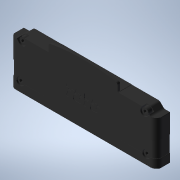
# Autodesk Inventor part: ETH2-17-L_2
Saved by Autodesk Inventor 2021 (Build 250183000, 183)
## iProperties
Created: 2025-05-01
Part Number: ETH2-17-L_2
Material: Generic
Catalog Web Link: www.cadenas.de
Description: ETH2_17_2-ETH2
Vendor: TOYO
Document SubType Name: Modeling
Designer: psAdmin
Manufacturer: TOYO
Mass: 101.271 g
Surface Area: 224.484 cm^2
Volume: 101.271 cm^3
Density: 1 g/cm^3
Appearance: PSOLRGB-175-175-175
Category: PARTsolutions
Company: TOYO
Title: ETH2-17-L
Author: Cadenas PARTsolutions
Comments: ETH2
PSOL_IDENT_0: {$CADENAS_DATA/23d-libs/toyo/eth2_series/eth2_17/parts/eth2_17_body2.prj},165 {VTYP=3D},{NB=ETH2-17-
PSOL_IDENT_1: L_2},{LINA=ETH2-17-L},{NN=ETH2_17_2},{DATE=02.07.2024 05:59:00},{GEOMDATE=07.06.2024 03:32:00},{VERS
PSOL_IDENT_2: ION=},{LINEID=10},{WBVAR=SD},{WBNUMERIC=}  {NB=ETH2-17-L_2},{LINA=ETH2-17-L},{KT=DUMMY},{CNSORDERNO=
PSOL_IDENT_3: ETH2-17-L},{MODEL=ETH2-17},{SD=L}
NB: ETH2-17-L_2
NN: ETH2_17_2
NT: ETH2
NBSYN: $CNSORDERNO._2
LINA: ETH2-17-L
CATALOG: TOYO
MODEL: ETH2-17
SD: L: Left side of slide
SUPPLIER: TOYO
ARTICLENO: ETH2-17-L_2
BOMINFO: ETH2-17-L
CREATOR: CADENAS GmbH
Autodesk Inventor part; units mm, degrees
sketch "__7" plane through (0, 0, 0) normal (0, 0, 1) x (1, 0, 0)
  arc A0 (-75.05, 41.2828) -> (-74.9914, 41.1414) centre (-74.85, 41.2828) ccw
  line L0 (-74.9914, 41.1414) -> (-74.6814, 40.8314)
  arc A1 (-73.8505, 39.5812) -> (-74.6814, 40.8314) centre (-77.3684, 38.1444) ccw
  line L1 (-73.8505, 39.5812) -> (-73.85, 39.58)
  line L2 (-73.85, 39.58) -> (-73.85, 35.42)
  line L3 (-73.85, 35.42) -> (-73.8505, 35.4188)
  arc A2 (-74.6814, 34.1686) -> (-73.8505, 35.4188) centre (-77.3684, 36.8556) ccw
  line L4 (-74.6814, 34.1686) -> (-74.9914, 33.8586)
  arc A3 (-74.9914, 33.8586) -> (-75.05, 33.7172) centre (-74.85, 33.7172) ccw
  line L5 (-75.05, 33.7172) -> (-75.05, 25.5)
  line L6 (-75.05, 25.5) -> (-74.55, 25)
  line L7 (-74.55, 25) -> (-74.55, 9)
  line L8 (-74.55, 9) -> (-75.05, 8.5)
  line L9 (-75.05, 8.5) -> (-75.05, 0.5)
  arc A4 (-75.05, 0.5) -> (-74.55, 0) centre (-74.55, 0.5) ccw
  line L10 (-74.55, 0) -> (74.55, 0)
  arc A5 (74.55, 0) -> (75.05, 0.5) centre (74.55, 0.5) ccw
  line L11 (75.05, 0.5) -> (75.05, 8.5)
  line L12 (75.05, 8.5) -> (74.55, 9)
  line L13 (74.55, 9) -> (74.55, 25)
  line L14 (74.55, 25) -> (75.05, 25.5)
  line L15 (75.05, 25.5) -> (75.05, 44.5)
  arc A6 (75.05, 44.5) -> (74.55, 45) centre (74.55, 44.5) ccw
  line L16 (74.55, 45) -> (70.2726, 45)
  arc A7 (68.1513, 45.8787) -> (70.2726, 45) centre (70.2726, 48) ccw
  line L17 (68.1513, 45.8787) -> (65.1087, 48.9213)
  arc A8 (65.1087, 48.9213) -> (62.9874, 49.8) centre (62.9874, 46.8) ccw
  line L18 (62.9874, 49.8) -> (36.13, 49.8)
  arc A9 (35.73, 50) -> (36.13, 49.8) centre (36.13, 50.3) ccw
  line L19 (35.73, 50) -> (35.24, 50)
  line L20 (35.24, 50) -> (35.24, 56.36)
  arc A10 (35.24, 56.36) -> (33.83, 58.08) centre (33.0401, 55.9946) ccw
  arc A11 (33.83, 58.08) -> (-33.83, 58.08) centre (0, -120.6057) ccw
  arc A12 (-33.83, 58.08) -> (-35.24, 56.36) centre (-33.0401, 55.9946) ccw
  line L21 (-35.24, 56.36) -> (-35.24, 50)
  line L22 (-35.24, 50) -> (-35.73, 50)
  arc A13 (-36.13, 49.8) -> (-35.73, 50) centre (-36.13, 50.3) ccw
  line L23 (-36.13, 49.8) -> (-62.9874, 49.8)
  arc A14 (-62.9874, 49.8) -> (-65.1087, 48.9213) centre (-62.9874, 46.8) ccw
  line L24 (-65.1087, 48.9213) -> (-68.1513, 45.8787)
  arc A15 (-70.2726, 45) -> (-68.1513, 45.8787) centre (-70.2726, 48) ccw
  line L25 (-70.2726, 45) -> (-74.55, 45)
  arc A16 (-74.55, 45) -> (-75.05, 44.5) centre (-74.55, 44.5) ccw
  line L26 (-75.05, 44.5) -> (-75.05, 41.2828)
  constraints: 54 end point, 34 point on circle, 17 centre point
extrude "Extrusion1" add sketch "__7" along normal blind 14
sketch "__2" plane through (0, 0, 0) normal (0, 1, 0) x (-1, 0, 0)
  line L0 (75.05, 8) -> (75.05, 15)
  line L1 (75.05, 15) -> (-75.05, 15)
  line L2 (-75.05, 15) -> (-75.05, 8)
  arc A0 (-69.05, 14) -> (-75.05, 8) centre (-69.05, 8) ccw
  line L3 (-69.05, 14) -> (69.05, 14)
  arc A1 (75.05, 8) -> (69.05, 14) centre (69.05, 8) ccw
  constraints: 8 end point, 4 point on circle, 2 centre point
extrude "Extrusion2" cut sketch "__2" along normal blind 49.33
sketch "__3" plane through (0, 16.76, 0) normal (0, 1, 0) x (1, 0, 0)
  line L0 (30.7, -14) -> (30.7, -18)
  line L1 (30.7, -18) -> (80, -18)
  line L2 (80, -18) -> (80, 0)
  line L3 (80, 0) -> (74.55, 0)
  line L4 (74.55, 0) -> (74.55, -8)
  arc A0 (69.05, -13.5) -> (74.55, -8) centre (69.05, -8) ccw
  line L5 (69.05, -13.5) -> (30.7, -14)
  constraints: 12 end point, 2 point on circle, 1 centre point
extrude "Extrusion3" cut sketch "__3" along normal mid plane 16
sketch "__4" plane through (0, 16.76, 0) normal (0, 1, 0) x (1, 0, 0)
  line L0 (-80, -18) -> (-30.7, -18)
  line L1 (-30.7, -18) -> (-30.7, -14)
  line L2 (-30.7, -14) -> (-69.05, -13.5)
  arc A0 (-74.55, -8) -> (-69.05, -13.5) centre (-69.05, -8) ccw
  line L3 (-74.55, -8) -> (-74.55, 0)
  line L4 (-74.55, 0) -> (-80, 0)
  line L5 (-80, 0) -> (-80, -18)
  constraints: 12 end point, 2 point on circle, 1 centre point
extrude "Extrusion4" cut sketch "__4" along normal mid plane 16
sketch "__6" plane through (0, 0, 14) normal (0, 0, 1) x (1, 0, 0)
  line L0 (-28.3226, 12.5645) -> (27.828, 12.5645)
  line L1 (27.828, 12.5645) -> (27.828, 38.9523)
  line L2 (27.828, 38.9523) -> (-28.3226, 38.9523)
  line L3 (-28.3226, 38.9523) -> (-28.3226, 12.5645)
  line L4 (13.552, 25.883) -> (16.452, 25.883)
  line L5 (16.452, 25.883) -> (16.567, 26.237)
  line L6 (16.567, 26.237) -> (13.666, 26.237)
  line L7 (13.666, 26.237) -> (13.552, 25.883)
  line L8 (8.386, 26.918) -> (11.328, 26.918)
  line L9 (11.328, 26.918) -> (11.778, 28.315)
  line L10 (11.778, 28.315) -> (14.296, 28.315)
  line L11 (14.296, 28.315) -> (13.846, 26.918)
  line L12 (13.846, 26.918) -> (16.788, 26.918)
  line L13 (16.788, 26.918) -> (17.326, 28.591)
  line L14 (17.326, 28.591) -> (17.578, 29.948)
  line L15 (17.578, 29.948) -> (17.189, 31.219)
  line L16 (17.189, 31.219) -> (16.218, 31.655)
  line L17 (16.218, 31.655) -> (11.516, 31.655)
  line L18 (11.516, 31.655) -> (10.052, 30.975)
  line L19 (10.052, 30.975) -> (9.344, 29.894)
  line L20 (9.344, 29.894) -> (8.386, 26.918)
  line L21 (8.092, 25.883) -> (10.992, 25.883)
  line L22 (10.992, 25.883) -> (11.107, 26.237)
  line L23 (11.107, 26.237) -> (8.207, 26.237)
  line L24 (8.207, 26.237) -> (8.092, 25.883)
  line L25 (7.048, 21.98) -> (7.502, 20.731)
  line L26 (7.502, 20.731) -> (8.495, 20.346)
  line L27 (8.495, 20.346) -> (13.197, 20.346)
  line L28 (13.197, 20.346) -> (14.512, 21.028)
  line L29 (14.512, 21.028) -> (15.163, 22.013)
  line L30 (15.163, 22.013) -> (16.178, 25.167)
  line L31 (16.178, 25.167) -> (13.278, 25.167)
  line L32 (13.278, 25.167) -> (12.828, 23.782)
  line L33 (12.828, 23.782) -> (10.31, 23.782)
  line L34 (10.31, 23.782) -> (10.76, 25.167)
  line L35 (10.76, 25.167) -> (7.859, 25.167)
  line L36 (7.859, 25.167) -> (7.164, 23.006)
  arc A0 (7.164, 23.006) -> (7.048, 21.98) centre (16.6662, 21.4121) ccw
  line L37 (1.608, 26.453) -> (1.68, 26.1)
  line L38 (1.68, 26.1) -> (5.124, 26.1)
  line L39 (5.124, 26.1) -> (5.415, 26.453)
  line L40 (5.415, 26.453) -> (1.608, 26.453)
  line L41 (0.637, 31.655) -> (1.482, 27.134)
  line L42 (1.482, 27.134) -> (5.962, 27.134)
  line L43 (5.962, 27.134) -> (9.701, 31.655)
  line L44 (9.701, 31.655) -> (6.617, 31.655)
  line L45 (6.617, 31.655) -> (4.123, 28.467)
  line L46 (4.123, 28.467) -> (3.637, 31.655)
  line L47 (3.637, 31.655) -> (0.637, 31.655)
  line L48 (0.214, 20.43) -> (2.891, 20.43)
  line L49 (2.891, 20.43) -> (4.484, 25.383)
  line L50 (4.484, 25.383) -> (1.808, 25.383)
  line L51 (1.808, 25.383) -> (0.214, 20.43)
  line L52 (-3.724, 25.883) -> (-0.824, 25.883)
  line L53 (-0.824, 25.883) -> (-0.709, 26.237)
  line L54 (-0.709, 26.237) -> (-3.609, 26.237)
  line L55 (-3.609, 26.237) -> (-3.724, 25.883)
  line L56 (-8.889, 26.918) -> (-5.947, 26.918)
  line L57 (-5.947, 26.918) -> (-5.498, 28.315)
  line L58 (-5.498, 28.315) -> (-2.98, 28.315)
  line L59 (-2.98, 28.315) -> (-3.429, 26.918)
  line L60 (-3.429, 26.918) -> (-0.487, 26.918)
  line L61 (-0.487, 26.918) -> (0.051, 28.591)
  line L62 (0.051, 28.591) -> (0.302, 29.948)
  line L63 (0.302, 29.948) -> (-0.086, 31.218)
  line L64 (-0.086, 31.218) -> (-1.057, 31.655)
  line L65 (-1.057, 31.655) -> (-5.759, 31.655)
  line L66 (-5.759, 31.655) -> (-7.223, 30.974)
  line L67 (-7.223, 30.974) -> (-7.932, 29.894)
  line L68 (-7.932, 29.894) -> (-8.889, 26.918)
  line L69 (-9.184, 25.883) -> (-6.283, 25.883)
  line L70 (-6.283, 25.883) -> (-6.169, 26.237)
  line L71 (-6.169, 26.237) -> (-9.069, 26.237)
  line L72 (-9.069, 26.237) -> (-9.184, 25.883)
  line L73 (-10.228, 21.98) -> (-9.773, 20.731)
  line L74 (-9.773, 20.731) -> (-8.781, 20.346)
  line L75 (-8.781, 20.346) -> (-4.079, 20.346)
  line L76 (-4.079, 20.346) -> (-2.763, 21.029)
  line L77 (-2.763, 21.029) -> (-2.112, 22.013)
  line L78 (-2.112, 22.013) -> (-1.098, 25.167)
  line L79 (-1.098, 25.167) -> (-3.998, 25.167)
  line L80 (-3.998, 25.167) -> (-4.448, 23.782)
  line L81 (-4.448, 23.782) -> (-6.966, 23.782)
  line L82 (-6.966, 23.782) -> (-6.516, 25.167)
  line L83 (-6.516, 25.167) -> (-9.416, 25.167)
  line L84 (-9.416, 25.167) -> (-10.112, 23.006)
  arc A1 (-10.112, 23.006) -> (-10.228, 21.98) centre (-0.6098, 21.4121) ccw
  line L85 (-15.678, 26.1) -> (-13.009, 26.1)
  line L86 (-13.009, 26.1) -> (-12.894, 26.453)
  line L87 (-12.894, 26.453) -> (-15.564, 26.453)
  line L88 (-15.564, 26.453) -> (-15.678, 26.1)
  line L89 (-17.533, 20.43) -> (-14.856, 20.43)
  line L90 (-14.856, 20.43) -> (-13.263, 25.383)
  line L91 (-13.263, 25.383) -> (-15.939, 25.383)
  line L92 (-15.939, 25.383) -> (-17.533, 20.43)
  line L93 (-17.608, 28.678) -> (-14.821, 28.678)
  line L94 (-14.821, 28.678) -> (-15.318, 27.134)
  line L95 (-15.318, 27.134) -> (-12.641, 27.134)
  line L96 (-12.641, 27.134) -> (-12.145, 28.678)
  line L97 (-12.145, 28.678) -> (-9.358, 28.678)
  line L98 (-9.358, 28.678) -> (-8.392, 31.655)
  line L99 (-8.392, 31.655) -> (-16.642, 31.655)
  line L100 (-16.642, 31.655) -> (-17.608, 28.678)
  constraints: 202 end point, 4 point on circle, 2 centre point
sketch "__5" plane through (0, 0, 14) normal (0, 0, 1) x (1, 0, 0)
  line L0 (-28.3226, 12.5645) -> (27.828, 12.5645)
  line L1 (27.828, 12.5645) -> (27.828, 38.9523)
  line L2 (27.828, 38.9523) -> (-28.3226, 38.9523)
  line L3 (-28.3226, 38.9523) -> (-28.3226, 12.5645)
  constraints: 8 end point
extrude "Extrusion5" cut sketch "__5" against normal blind 0.49
extrude "Extrusion6" add sketch "__6" against normal blind 0.49
sketch "__8" plane through (0, 0, 0) normal (0, 1, 0) x (-1, 0, 0)
  arc A0 (55, 6) -> (61, 0) centre (61, 6) ccw
  line L0 (55, 6) -> (55, 10.5)
  line L1 (55, 10.5) -> (-55, 10.5)
  line L2 (-55, 10.5) -> (-55, 6)
  arc A1 (-61, 0) -> (-55, 6) centre (-61, 6) ccw
  line L3 (-61, 0) -> (61, 0)
  constraints: 8 end point, 4 point on circle, 2 centre point
extrude "Extrusion7" cut sketch "__8" along normal blind 2
sketch "__9" plane through (0, 0, 0) normal (0, 0, 1) x (1, 0, 0)
  line L0 (-35.24, 56.56) -> (-35.24, 50)
  line L1 (-35.24, 50) -> (35.24, 50)
  line L2 (35.24, 50) -> (35.24, 56.56)
  arc A0 (35.24, 56.56) -> (33.83, 58.08) centre (33.0875, 55.9772) ccw
  arc A1 (33.83, 58.08) -> (-33.83, 58.08) centre (0, -120.6057) ccw
  arc A2 (-33.83, 58.08) -> (-35.24, 56.56) centre (-33.0875, 55.9772) ccw
  constraints: 6 end point, 6 point on circle, 3 centre point
extrude "Extrusion8" cut sketch "__9" along normal blind 11.43
sketch "__10" plane through (0, 0, 14) normal (0, 0, 1) x (1, 0, 0)
  arc A0 (58.9765, 47.6534) -> (65.5534, 43.1761) centre (62.5, 45.76) ccw
  line L0 (65.5534, 43.1761) -> (67.74, 45.76)
  line L1 (67.74, 45.76) -> (67.74, 50)
  line L2 (67.74, 50) -> (60.13, 49.8)
  line L3 (60.13, 49.8) -> (58.9765, 47.6534)
  constraints: 8 end point, 2 point on circle, 1 centre point
extrude "Extrusion9" cut sketch "__10" against normal blind 5
sketch "__11" plane through (0, 0, 14) normal (0, 0, 1) x (1, 0, 0)
  line L0 (-67.74, 50) -> (-67.74, 45.76)
  line L1 (-67.74, 45.76) -> (-65.5534, 43.1761)
  arc A0 (-65.5534, 43.1761) -> (-58.9765, 47.6534) centre (-62.5, 45.76) ccw
  line L2 (-58.9765, 47.6534) -> (-60.13, 49.8)
  line L3 (-60.13, 49.8) -> (-67.74, 50)
  constraints: 8 end point, 2 point on circle, 1 centre point
extrude "Extrusion10" cut sketch "__11" against normal blind 5
sketch "__12" plane through (0, 0, 14) normal (0, 0, 1) x (1, 0, 0)
  circle A0 centre (64.5, 9.5) radius 4
  constraints: 1 centre point
extrude "Extrusion11" cut sketch "__12" against normal blind 5
sketch "__13" plane through (0, 0, 14) normal (0, 0, 1) x (1, 0, 0)
  circle A0 centre (-64.5, 9.5) radius 4
  constraints: 1 centre point
extrude "Extrusion12" cut sketch "__13" against normal blind 5
sketch "__14" plane through (62.5, 45.76, 9) normal (0, 0, 1) x (1, 0, 0)
  circle A0 centre (0, 0) radius 3.5
  constraints: 1 centre point
extrude "Extrusion13" add sketch "__14" along normal blind 4
sketch "Pattern_1_SKETCH_1" plane through (0, 0, 9) normal (0, 0, 1) x (1, 0, 0)
  circle A0 centre (-62.5, 45.76) radius 3.5
  constraints: 1 centre point
sketch "Pattern_1_SKETCH_2" plane through (0, 0, 9) normal (0, 0, 1) x (1, 0, 0)
  circle A0 centre (64.5, 9.5) radius 3.5
  constraints: 1 centre point
sketch "Pattern_1_SKETCH_3" plane through (0, 0, 9) normal (0, 0, 1) x (1, 0, 0)
  circle A0 centre (-64.5, 9.5) radius 3.5
  constraints: 1 centre point
extrude "Extrusion14" add sketch "Pattern_1_SKETCH_1" along normal blind 4
extrude "Extrusion15" add sketch "Pattern_1_SKETCH_2" along normal blind 4
extrude "Extrusion16" add sketch "Pattern_1_SKETCH_3" along normal blind 4
sketch "__16" plane through (62.5, 45.76, 13) normal (0, 0, 1) x (1, 0, 0)
  line L0 (-1.7321, 0) -> (-0.866, -1.5)
  line L1 (-0.866, -1.5) -> (0.866, -1.5)
  line L2 (0.866, -1.5) -> (1.7321, 0)
  line L3 (1.7321, 0) -> (0.866, 1.5)
  line L4 (0.866, 1.5) -> (-0.866, 1.5)
  line L5 (-0.866, 1.5) -> (-1.7321, 0)
  constraints: 12 end point
extrude "Extrusion17" cut sketch "__16" against normal blind 2
sketch "Pattern_2_SKETCH_1" plane through (0, 0, 13) normal (0, 0, 1) x (1, 0, 0)
  line L0 (-64.2321, 45.76) -> (-63.366, 44.26)
  line L1 (-63.366, 44.26) -> (-61.634, 44.26)
  line L2 (-61.634, 44.26) -> (-60.7679, 45.76)
  line L3 (-60.7679, 45.76) -> (-61.634, 47.26)
  line L4 (-61.634, 47.26) -> (-63.366, 47.26)
  line L5 (-63.366, 47.26) -> (-64.2321, 45.76)
  constraints: 12 end point
sketch "Pattern_2_SKETCH_2" plane through (0, 0, 13) normal (0, 0, 1) x (1, 0, 0)
  line L0 (62.7679, 9.5) -> (63.634, 8)
  line L1 (63.634, 8) -> (65.366, 8)
  line L2 (65.366, 8) -> (66.2321, 9.5)
  line L3 (66.2321, 9.5) -> (65.366, 11)
  line L4 (65.366, 11) -> (63.634, 11)
  line L5 (63.634, 11) -> (62.7679, 9.5)
  constraints: 12 end point
sketch "Pattern_2_SKETCH_3" plane through (0, 0, 13) normal (0, 0, 1) x (1, 0, 0)
  line L0 (-66.2321, 9.5) -> (-65.366, 8)
  line L1 (-65.366, 8) -> (-63.634, 8)
  line L2 (-63.634, 8) -> (-62.7679, 9.5)
  line L3 (-62.7679, 9.5) -> (-63.634, 11)
  line L4 (-63.634, 11) -> (-65.366, 11)
  line L5 (-65.366, 11) -> (-66.2321, 9.5)
  constraints: 12 end point
extrude "Extrusion18" cut sketch "Pattern_2_SKETCH_1" against normal blind 2
extrude "Extrusion19" cut sketch "Pattern_2_SKETCH_2" against normal blind 2
extrude "Extrusion20" cut sketch "Pattern_2_SKETCH_3" against normal blind 2
ref_plane "BODYY_XY" through (0, 0, 10.5) normal (0, 0, 1) x (1, 0, 0)
ref_plane "BODYY_YZ" through (0, 0, 10.5) normal (1, 0, 0) x (0, 1, 0)
ref_plane "BODYY_ZX" through (0, 0, 10.5) normal (0, 1, 0) x (0, 0, 1)
body "Solid1"
